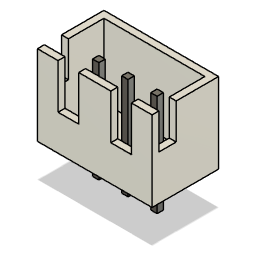
XH 2.54mm 3pin connector (Autodesk Fusion 360 design; units mm, degrees)
Autodesk Fusion 360 part; units mm, degrees
sketch "Sketch1" plane through (0, 0, 0) normal (0, 1, 0) x (1, 0, 0)
  line L0 (5, -2.9) -> (-5, -2.9)
  line L1 (-5, -2.9) -> (-5, 2.9)
  line L2 (-5, 2.9) -> (5, 2.9)
  line L3 (5, 2.9) -> (5, -2.9)
  line L4 (5, -2.9) -> (-5, 2.9) construction
  line L5 (-5, -2.9) -> (5, 2.9) construction
  line L6 (4.4, -2.3) -> (-4.4, -2.3)
  line L7 (-4.4, -2.3) -> (-4.4, 2.3)
  line L8 (-4.4, 2.3) -> (4.4, 2.3)
  line L9 (4.4, 2.3) -> (4.4, -2.3)
  dimension "d1" = 10
  dimension "d2" = 5.8
  dimension "d3" = 0.6
  constraint horizontal L0
  constraint perpendicular L0 L1
  constraint parallel L0 L2
  constraint parallel L1 L3
  constraint coincident L4 origin
  constraint coincident L5 origin
  measures "d1" distance of L1.end L2.end
  measures "d2" distance of L0.end L1.end
extrude "Extrude1" add sketch "Sketch1" along normal blind 0.6 contours L6 L7 L8 L9 makes body 1
extrude "Extrude2" add sketch "Sketch1" along normal blind 7 bodies 1
sketch "Sketch2" plane through (0, 0, 2.9) normal (0, 0, 1) x (1, 0, 0)
  line L0 (-5, 0) -> (5, 0)
  line L1 (5, 0) -> (5, 7)
  line L2 (5, 7) -> (-5, 7)
  line L3 (-5, 7) -> (-5, 0)
  line L4 (5, 7) -> (3.2, 7) construction
  line L5 (-5, 7) -> (-3.2, 7) construction
  line L6 (-3.2, 7) -> (-3.2, 3.1)
  line L7 (-3.2, 3.1) -> (-1.4, 3.1)
  line L8 (-1.4, 3.1) -> (-1.4, 7)
  line L9 (-1.4, 3.1) -> (5, 3.1) construction
  line L10 (3.2, 7) -> (3.2, 3.1)
  line L11 (3.2, 3.1) -> (1.4, 3.1)
  line L12 (1.4, 3.1) -> (1.4, 7.0013)
  dimension "d8" = 1.8
  dimension "d9" = 1.8
  dimension "d10" = 3.9
  dimension "d11" = 1.8
  dimension "d12" = 90
  dimension "d13" = 1.8
  dimension "d14" = 90
  constraint coincident L1.end L2.start
  constraint perpendicular L1 L4
  constraint coincident L2.end L3.start
  constraint perpendicular L3 L5
  constraint perpendicular L5 L6
  constraint perpendicular L6 L7
  constraint coincident L2 L8.end
  constraint coincident L1 L9.end
  constraint perpendicular L1 L9
  constraint coincident L9 L10.end
  constraint perpendicular L9 L10
  constraint perpendicular L10 L11
  measures "d8" distance of L1.end L4.end
  measures "d9" distance of L2.end L5.end
  measures "d10" distance of L5.end L6.end
  measures "d11" distance of L6.end L7.end
  measures "d12" angle of L7 L8
  measures "d13" distance of L10.end L11.end
  measures "d14" angle of L11 L12
extrude "Extrude3" cut sketch "Sketch2" against normal blind 1 contours L2 L6 L7 L8 | L2 L10 L11 L12 bodies 1
sketch "Sketch3" plane through (5, 0, 0) normal (1, 0, 0) x (0, 0, -1)
  line L0 (-2.9, 0) -> (2.9, 0)
  line L1 (2.9, 0) -> (2.9, 7)
  line L2 (2.9, 7) -> (-2.9, 7)
  line L3 (-2.9, 7) -> (-2.9, 0)
  line L4 (-2.3, 7) -> (-2.3, 3.9)
  line L5 (-2.3, 3.9) -> (-0.8, 3.9)
  line L6 (-0.8, 3.9) -> (-0.8, 7)
  point P0 (-2.3, 7)
  dimension "d17" = 3.1
  dimension "d18" = 1.5
  dimension "d19" = 90
  constraint coincident P0 L4.start
  constraint perpendicular L2 L4
  constraint perpendicular L4 L5
  constraint coincident L2 L6.end
  measures "d17" distance of P0 L4.end
  measures "d18" distance of L4.end L5.end
  measures "d19" angle of L5 L6
extrude "Extrude4" cut sketch "Sketch3" against normal blind 13.5 contours L2 L4 L5 L6 bodies 1
sketch "Sketch4" plane through (0, 0, 0) normal (0, -1, 0) x (1, 0, 0)
  line L0 (-5, -2.9) -> (5, -2.9)
  line L1 (5, -2.9) -> (5, 2.9)
  line L2 (5, 2.9) -> (-5, 2.9)
  line L3 (-5, 2.9) -> (-5, -2.9)
  line L4 (0.275, -0.275) -> (-0.275, -0.275)
  line L5 (-0.275, -0.275) -> (-0.275, 0.275)
  line L6 (-0.275, 0.275) -> (0.275, 0.275)
  line L7 (0.275, 0.275) -> (0.275, -0.275)
  line L8 (0.275, -0.275) -> (-0.275, 0.275) construction
  line L9 (-0.275, -0.275) -> (0.275, 0.275) construction
  line L10 (0, 0) -> (2.54, 0) construction
  line L11 (0, 0) -> (-2.54, 0) construction
  line L12 (-2.265, -0.275) -> (-2.815, -0.275)
  line L13 (-2.815, -0.275) -> (-2.815, 0.275)
  line L14 (-2.815, 0.275) -> (-2.265, 0.275)
  line L15 (-2.265, 0.275) -> (-2.265, -0.275)
  line L16 (-2.265, -0.275) -> (-2.815, 0.275) construction
  line L17 (-2.815, -0.275) -> (-2.265, 0.275) construction
  line L18 (2.815, -0.275) -> (2.265, -0.275)
  line L19 (2.265, -0.275) -> (2.265, 0.275)
  line L20 (2.265, 0.275) -> (2.815, 0.275)
  line L21 (2.815, 0.275) -> (2.815, -0.275)
  line L22 (2.815, -0.275) -> (2.265, 0.275) construction
  line L23 (2.265, -0.275) -> (2.815, 0.275) construction
  point P0 (-2.54, 0)
  point P1 (2.54, 0)
  dimension "d22" = 0.55
  dimension "d23" = 0.55
  dimension "d24" = 2.54
  dimension "d25" = 2.54
  dimension "d26" = 0.55
  dimension "d27" = 0.55
  dimension "d28" = 0.55
  dimension "d29" = 0.55
  constraint horizontal L4
  constraint perpendicular L4 L5
  constraint parallel L4 L6
  constraint parallel L5 L7
  constraint coincident L8 L10.start
  constraint coincident L9 L10.start
  constraint coincident L10.start L11.start
  constraint perpendicular L7 L10
  constraint perpendicular L5 L11
  constraint horizontal L12
  constraint perpendicular L12 L13
  constraint parallel L12 L14
  constraint parallel L13 L15
  constraint coincident L16 P0
  constraint coincident L17 P0
  constraint coincident P0 L11.end
  constraint horizontal L18
  constraint perpendicular L18 L19
  constraint parallel L18 L20
  constraint parallel L19 L21
  constraint coincident L22 P1
  constraint coincident L23 P1
  constraint coincident P1 L10.end
  measures "d22" distance of L5.end L6.end
  measures "d23" distance of L4.end L5.end
  measures "d24" distance of L10.start P1
  measures "d25" distance of L10.start P0
  measures "d26" distance of L13.end L14.end
  measures "d27" distance of L12.end L13.end
  measures "d28" distance of L19.end L20.end
  measures "d29" distance of L18.end L19.end
extrude "Extrude5" cut sketch "Sketch4" against normal blind 1 contours L4 L5 L6 L7 | L12 L13 L14 L15 | L18 L19 L20 L21 bodies 1
extrude "Extrude6" add sketch "Sketch4" along normal blind 2.87 and the other way blind 6 separate body contours L4 L5 L6 L7 | L12 L13 L14 L15 | L18 L19 L20 L21 makes body 2 at (2.815, 0.0867, -0.0917) makes body 3 at (-0.0917, 0.0867, -0.275) makes body 4 at (-2.265, 0.0867, -0.0917)
